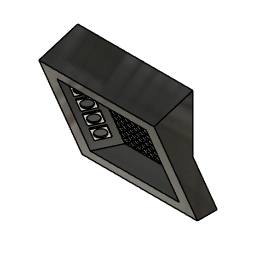
Face (Autodesk Fusion 360 design; units mm, degrees)
Autodesk Fusion 360 part; units mm, degrees
(part 1 of 2)
sketch "Sketch1" plane through (0, 0, 0) normal (0, 1, 0) x (1, 0, 0)
  line L0 (44, 44) -> (-44, 44)
  line L1 (-44, 44) -> (-44, -44)
  line L2 (-44, -44) -> (44, -44)
  line L3 (44, -44) -> (44, 44)
  line L4 (44, 44) -> (-44, -44) construction
  line L5 (-44, 44) -> (44, -44) construction
  dimension "d1" = 88
  dimension "d2" = 88
  constraint horizontal L0
  constraint perpendicular L0 L1
  constraint parallel L0 L2
  constraint parallel L1 L3
  constraint coincident L4 origin
  constraint coincident L5 origin
  measures "d1" distance of L1.end L2.end
  measures "d2" distance of L0.end L1.end
extrude "Extrude1" add sketch "Sketch1" along normal blind 31
sketch "Sketch2" plane through (44, 0, 0) normal (1, 0, 0) x (0, 1, 0)
  line L0 (0, 44) -> (0, -44)
  line L1 (0, -44) -> (31, -44)
  line L2 (31, -44) -> (31, 44)
  line L3 (31, 44) -> (0, 44)
  line L4 (31, 44) -> (31, 0)
  line L5 (31, 0) -> (49.4592, -44)
  line L6 (49.4592, -44) -> (34.4592, -44)
  line L7 (31, 44) -> (1.3859, 34.8347)
  line L8 (1.3859, 34.8347) -> (34.4592, -44)
  dimension "d5" = 15
  dimension "d6" = 31
  constraint coincident L2.end L3.start
  constraint midpoint L2 L4.end
  constraint perpendicular L2 L6
  constraint parallel L5 L8
  constraint collinear L1 L6
  measures "d5" distance of L5.end L6.end
  measures "d6" distance of L2.end L7.end
extrude "Extrude2" cut sketch "Sketch2" against normal blind 88 contours L0 L1 L2 L3 L7 L8
extrude "Extrude3" add sketch "Sketch2" against normal blind 88 contours L2 L5 L6 L8
sketch "Sketch3" plane through (0, 13.6054, 5.7078) normal (0, -0.922137, -0.386863) x (1, 0, 0)
  line L0 (44, -53.905) -> (44, 31.5863)
  line L1 (44, 31.5863) -> (-44, 31.5863)
  line L2 (-44, 31.5863) -> (-44, -53.905)
  line L3 (-44, -53.905) -> (44, -53.905)
  line L4 (34, -43.905) -> (34, 21.5863)
  line L5 (34, 21.5863) -> (-34, 21.5863)
  line L6 (-34, 21.5863) -> (-34, -43.905)
  line L7 (-34, -43.905) -> (34, -43.905)
  dimension "d11" = -10
extrude "Extrude4" cut sketch "Sketch3" against normal blind 80 contours L4 L5 L6 L7
sketch "Sketch4" plane through (0, 16.9852, -40.4865) normal (0, -0.386863, 0.922137) x (1, 0, 0)
  line L0 (34, 28.5863) -> (-34, 28.5863)
  line L1 (-34, 28.5863) -> (-34, 14.7542)
  line L2 (-34, 14.7542) -> (34, 14.7542)
  line L3 (34, 14.7542) -> (34, 28.5863)
  line L4 (-34, 14.7542) -> (-20.1679, 28.5863)
  line L5 (-34, 14.7542) -> (-19.9723, 14.7542) construction
  line L6 (-20.1679, 28.5863) -> (-34, 28.5863)
  line L7 (34, 14.7542) -> (20.1679, 28.5863)
  line L8 (34, 14.7542) -> (60.9464, 14.7542) construction
  line L9 (20.1679, 28.5863) -> (34, 28.5863)
  dimension "d14" = 45
  dimension "d15" = 135
  constraint horizontal L5
  constraint coincident L1.end L2.start
  constraint coincident L0 L4.end
  constraint coincident L0.end L1.start
  constraint horizontal L8
  constraint coincident L2.end L3.start
  constraint coincident L0.start L3.end
  constraint collinear L0 L9
  measures "d14" angle of L4 L5
  measures "d15" angle of L7 L8
extrude "Extrude5" add sketch "Sketch4" along normal up to surface (65.4913 mm away) contours L0 L3 L7 L9 | L0 L1 L4 L6
sketch "Sketch5" plane through (-24.3771, 22.479, 9.4306) normal (0.707107, -0.65205, -0.273553) x (0.677907, 0.735148, 0)
  line L0 (-0.4323, 22.3878) -> (-19.186, 16.8245)
  line L1 (-19.186, 16.8245) -> (-0.5602, -45.9624)
  line L2 (-0.5602, -45.9624) -> (18.1935, -40.3991)
  line L3 (18.1935, -40.3991) -> (-0.4323, 22.3878)
  line L4 (-9.8092, 19.6062) -> (8.8166, -43.1807) construction
  circle A0 centre (4.835, -29.7588) radius 4
  line L5 (-1.3805, -26.3873) -> (8.2065, -23.5433)
  line L6 (8.2065, -23.5433) -> (11.0505, -33.1304)
  line L7 (11.0505, -33.1304) -> (1.4635, -35.9744)
  line L8 (1.4635, -35.9744) -> (-1.3805, -26.3873)
  circle A1 centre (1.043, -16.9761) radius 4
  line L9 (-5.1725, -13.6046) -> (4.4145, -10.7606)
  line L10 (4.4145, -10.7606) -> (7.2585, -20.3476)
  line L11 (7.2585, -20.3476) -> (-2.3285, -23.1916)
  line L12 (-2.3285, -23.1916) -> (-5.1725, -13.6046)
  circle A2 centre (-2.749, -4.1934) radius 4
  line L13 (-8.9646, -0.8218) -> (0.6225, 2.0222)
  line L14 (0.6225, 2.0222) -> (3.4665, -7.5649)
  line L15 (3.4665, -7.5649) -> (-6.1205, -10.4089)
  line L16 (-6.1205, -10.4089) -> (-8.9646, -0.8218)
  circle A3 centre (-6.541, 8.5894) radius 4
  line L17 (-12.7566, 11.9609) -> (-3.1695, 14.8049)
  line L18 (-3.1695, 14.8049) -> (-0.3255, 5.2179)
  line L19 (-0.3255, 5.2179) -> (-9.9126, 2.3739)
  line L20 (-9.9126, 2.3739) -> (-12.7566, 11.9609)
  dimension "d18" = 8
  dimension "d19" = 10
  dimension "d20" = 10
  dimension "d21" = 5
  dimension "d22" = 5
  dimension "d23" = 14
  dimension "d26" = -40
  dimension "d27" = 0
  constraint midpoint L0 L4.start
  constraint midpoint L2 L4.end
  constraint coincident L4 A0.centre
  constraint perpendicular L5 L6
  constraint parallel L5 L7
  constraint parallel L6 L8
  constraint parallel L2 L7
  measures "d18" diameter of A0
  measures "d19" distance of L5.end L6.end
  measures "d20" distance of L6.end L7.end
  measures "d21" distance of A0.centre L6
  measures "d22" distance of A0.centre L7
  measures "d23" distance of L4.end A0.centre
extrude "Extrude6" add sketch "Sketch5" along normal blind 1 contours L5 L6 L7 L8 | L9 L10 L11 L12 | L13 L14 L15 L16 | L17 L18 L19 L20
mirror "Mirror1" about plane through (0, 0, 0) normal (1, 0, 0) of "Extrude6"
sketch "Sketch6" plane through (0, 26.3605, 11.059) normal (0, 0.922137, 0.386863) x (-1, 0, 0)
  line L0 (-34, -11.9927) -> (-44, -11.9927)
  line L1 (-44, -11.9927) -> (-44, -59.708)
  line L2 (-44, -59.708) -> (44, -59.708)
  line L3 (44, -59.708) -> (44, -11.9927)
  line L4 (44, -11.9927) -> (34, -11.9927)
  line L5 (34, -11.9927) -> (34, 21.5863)
  line L6 (34, 21.5863) -> (20.1679, 21.5863)
  line L7 (20.1679, 21.5863) -> (20.1679, -43.905)
  line L8 (20.1679, -43.905) -> (-20.1679, -43.905)
  line L9 (-20.1679, -43.905) -> (-20.1679, 21.5863)
  line L10 (-20.1679, 21.5863) -> (-34, 21.5863)
  line L11 (-34, 21.5863) -> (-34, -11.9927)
  line L12 (-27.084, 21.5863) -> (32.8322, 21.5863)
  line L13 (32.8322, 21.5863) -> (32.8322, -55.186)
  line L14 (32.8322, -55.186) -> (-27.084, -55.186)
  line L15 (-27.084, -55.186) -> (-27.084, 21.5863)
  line L16 (-27, -51.1716) -> (-28.1716, -50)
  line L17 (-28.1716, -50) -> (-29.8284, -50)
  line L18 (-29.8284, -50) -> (-31, -51.1716)
  line L19 (-31, -51.1716) -> (-31, -52.8284)
  line L20 (-31, -52.8284) -> (-29.8284, -54)
  line L21 (-29.8284, -54) -> (-28.1716, -54)
  line L22 (-28.1716, -54) -> (-27, -52.8284)
  line L23 (-27, -52.8284) -> (-27, -51.1716)
  line L24 (-29.8284, -49) -> (-28.1716, -49)
  line L25 (-28.1716, -45) -> (-29.8284, -45)
  line L26 (-28.1716, -49) -> (-27, -47.8284)
  line L27 (-31, -47.8284) -> (-29.8284, -49)
  line L28 (-31, -46.1716) -> (-31, -47.8284)
  line L29 (-27, -47.8284) -> (-27, -46.1716)
  line L30 (-29.8284, -45) -> (-31, -46.1716)
  line L31 (-27, -46.1716) -> (-28.1716, -45)
  line L32 (-29.8284, -44) -> (-28.1716, -44)
  line L33 (-28.1716, -40) -> (-29.8284, -40)
  line L34 (-28.1716, -44) -> (-27, -42.8284)
  line L35 (-31, -42.8284) -> (-29.8284, -44)
  line L36 (-31, -41.1716) -> (-31, -42.8284)
  line L37 (-27, -42.8284) -> (-27, -41.1716)
  line L38 (-29.8284, -40) -> (-31, -41.1716)
  line L39 (-27, -41.1716) -> (-28.1716, -40)
  line L40 (-29.8284, -39) -> (-28.1716, -39)
  line L41 (-28.1716, -35) -> (-29.8284, -35)
  line L42 (-28.1716, -39) -> (-27, -37.8284)
  line L43 (-31, -37.8284) -> (-29.8284, -39)
  line L44 (-31, -36.1716) -> (-31, -37.8284)
  line L45 (-27, -37.8284) -> (-27, -36.1716)
  line L46 (-29.8284, -35) -> (-31, -36.1716)
  line L47 (-27, -36.1716) -> (-28.1716, -35)
  line L48 (-29.8284, -34) -> (-28.1716, -34)
  line L49 (-28.1716, -30) -> (-29.8284, -30)
  line L50 (-28.1716, -34) -> (-27, -32.8284)
  line L51 (-31, -32.8284) -> (-29.8284, -34)
  line L52 (-31, -31.1716) -> (-31, -32.8284)
  line L53 (-27, -32.8284) -> (-27, -31.1716)
  line L54 (-29.8284, -30) -> (-31, -31.1716)
  line L55 (-27, -31.1716) -> (-28.1716, -30)
  line L56 (-29.8284, -29) -> (-28.1716, -29)
  line L57 (-28.1716, -25) -> (-29.8284, -25)
  line L58 (-28.1716, -29) -> (-27, -27.8284)
  line L59 (-31, -27.8284) -> (-29.8284, -29)
  line L60 (-31, -26.1716) -> (-31, -27.8284)
  line L61 (-27, -27.8284) -> (-27, -26.1716)
  line L62 (-29.8284, -25) -> (-31, -26.1716)
  line L63 (-27, -26.1716) -> (-28.1716, -25)
  line L64 (-29.8284, -24) -> (-28.1716, -24)
  line L65 (-28.1716, -20) -> (-29.8284, -20)
  line L66 (-28.1716, -24) -> (-27, -22.8284)
  line L67 (-31, -22.8284) -> (-29.8284, -24)
  line L68 (-31, -21.1716) -> (-31, -22.8284)
  line L69 (-27, -22.8284) -> (-27, -21.1716)
  line L70 (-29.8284, -20) -> (-31, -21.1716)
  line L71 (-27, -21.1716) -> (-28.1716, -20)
  line L72 (-29.8284, -19) -> (-28.1716, -19)
  line L73 (-28.1716, -15) -> (-29.8284, -15)
  line L74 (-28.1716, -19) -> (-27, -17.8284)
  line L75 (-31, -17.8284) -> (-29.8284, -19)
  line L76 (-31, -16.1716) -> (-31, -17.8284)
  line L77 (-27, -17.8284) -> (-27, -16.1716)
  line L78 (-29.8284, -15) -> (-31, -16.1716)
  line L79 (-27, -16.1716) -> (-28.1716, -15)
  line L80 (-29.8284, -14) -> (-28.1716, -14)
  line L81 (-28.1716, -10) -> (-29.8284, -10)
  line L82 (-28.1716, -14) -> (-27, -12.8284)
  line L83 (-31, -12.8284) -> (-29.8284, -14)
  line L84 (-31, -11.1716) -> (-31, -12.8284)
  line L85 (-27, -12.8284) -> (-27, -11.1716)
  line L86 (-29.8284, -10) -> (-31, -11.1716)
  line L87 (-27, -11.1716) -> (-28.1716, -10)
  line L88 (-29.8284, -9) -> (-28.1716, -9)
  line L89 (-28.1716, -5) -> (-29.8284, -5)
  line L90 (-28.1716, -9) -> (-27, -7.8284)
  line L91 (-31, -7.8284) -> (-29.8284, -9)
  line L92 (-31, -6.1716) -> (-31, -7.8284)
  line L93 (-27, -7.8284) -> (-27, -6.1716)
  line L94 (-29.8284, -5) -> (-31, -6.1716)
  line L95 (-27, -6.1716) -> (-28.1716, -5)
  line L96 (-29.8284, -4) -> (-28.1716, -4)
  line L97 (-28.1716, 0) -> (-29.8284, 0)
  line L98 (-28.1716, -4) -> (-27, -2.8284)
  line L99 (-31, -2.8284) -> (-29.8284, -4)
  line L100 (-31, -1.1716) -> (-31, -2.8284)
  line L101 (-27, -2.8284) -> (-27, -1.1716)
  line L102 (-29.8284, 0) -> (-31, -1.1716)
  line L103 (-27, -1.1716) -> (-28.1716, 0)
  line L104 (-29.8284, 1) -> (-28.1716, 1)
  line L105 (-28.1716, 5) -> (-29.8284, 5)
  line L106 (-28.1716, 1) -> (-27, 2.1716)
  line L107 (-31, 2.1716) -> (-29.8284, 1)
  line L108 (-31, 3.8284) -> (-31, 2.1716)
  line L109 (-27, 2.1716) -> (-27, 3.8284)
  line L110 (-29.8284, 5) -> (-31, 3.8284)
  line L111 (-27, 3.8284) -> (-28.1716, 5)
  line L112 (-29.8284, 6) -> (-28.1716, 6)
  line L113 (-28.1716, 10) -> (-29.8284, 10)
  line L114 (-28.1716, 6) -> (-27, 7.1716)
  line L115 (-31, 7.1716) -> (-29.8284, 6)
  line L116 (-31, 8.8284) -> (-31, 7.1716)
  line L117 (-27, 7.1716) -> (-27, 8.8284)
  line L118 (-29.8284, 10) -> (-31, 8.8284)
  line L119 (-27, 8.8284) -> (-28.1716, 10)
  line L120 (-29.8284, 11) -> (-28.1716, 11)
  line L121 (-28.1716, 15) -> (-29.8284, 15)
  line L122 (-28.1716, 11) -> (-27, 12.1716)
  line L123 (-31, 12.1716) -> (-29.8284, 11)
  line L124 (-31, 13.8284) -> (-31, 12.1716)
  line L125 (-27, 12.1716) -> (-27, 13.8284)
  line L126 (-29.8284, 15) -> (-31, 13.8284)
  line L127 (-27, 13.8284) -> (-28.1716, 15)
  line L128 (-29.8284, 16) -> (-28.1716, 16)
  line L129 (-28.1716, 20) -> (-29.8284, 20)
  line L130 (-28.1716, 16) -> (-27, 17.1716)
  line L131 (-31, 17.1716) -> (-29.8284, 16)
  line L132 (-31, 18.8284) -> (-31, 17.1716)
  line L133 (-27, 17.1716) -> (-27, 18.8284)
  line L134 (-29.8284, 20) -> (-31, 18.8284)
  line L135 (-27, 18.8284) -> (-28.1716, 20)
  line L136 (-26.0833, -6.1716) -> (-26.0833, -7.8284)
  line L137 (-23.2549, -40) -> (-24.9118, -40)
  line L138 (-22.0833, -27.8284) -> (-22.0833, -26.1716)
  line L139 (-24.9118, 5) -> (-26.0833, 3.8284)
  line L140 (-26.0833, -31.1716) -> (-26.0833, -32.8284)
  line L141 (-22.0833, -2.8284) -> (-22.0833, -1.1716)
  line L142 (-24.9118, 20) -> (-26.0833, 18.8284)
  line L143 (-26.0833, 2.1716) -> (-24.9118, 1)
  line L144 (-26.0833, -1.1716) -> (-26.0833, -2.8284)
  line L145 (-26.0833, 18.8284) -> (-26.0833, 17.1716)
  line L146 (-24.9118, -29) -> (-23.2549, -29)
  line L147 (-23.2549, -49) -> (-22.0833, -47.8284)
  line L148 (-23.2549, 5) -> (-24.9118, 5)
  line L149 (-23.2549, -24) -> (-22.0833, -22.8284)
  line L150 (-26.0833, -51.1716) -> (-26.0833, -52.8284)
  line L151 (-22.0833, -6.1716) -> (-23.2549, -5)
  line L152 (-22.0833, -47.8284) -> (-22.0833, -46.1716)
  line L153 (-22.0833, -32.8284) -> (-22.0833, -31.1716)
  line L154 (-22.0833, 8.8284) -> (-23.2549, 10)
  line L155 (-26.0833, 17.1716) -> (-24.9118, 16)
  line L156 (-24.9118, -9) -> (-23.2549, -9)
  line L157 (-22.0833, -46.1716) -> (-23.2549, -45)
  line L158 (-23.2549, 16) -> (-22.0833, 17.1716)
  line L159 (-23.2549, -44) -> (-22.0833, -42.8284)
  line L160 (-24.9118, -14) -> (-23.2549, -14)
  line L161 (-23.2549, 6) -> (-22.0833, 7.1716)
  line L162 (-24.9118, -49) -> (-23.2549, -49)
  line L163 (-24.9118, -44) -> (-23.2549, -44)
  line L164 (-22.0833, -21.1716) -> (-23.2549, -20)
  line L165 (-24.9118, 1) -> (-23.2549, 1)
  line L166 (-23.2549, -4) -> (-22.0833, -2.8284)
  line L167 (-22.0833, -17.8284) -> (-22.0833, -16.1716)
  line L168 (-23.2549, -30) -> (-24.9118, -30)
  line L169 (-24.9118, -5) -> (-26.0833, -6.1716)
  line L170 (-23.2549, -19) -> (-22.0833, -17.8284)
  line L171 (-23.2549, -14) -> (-22.0833, -12.8284)
  line L172 (-26.0833, -22.8284) -> (-24.9118, -24)
  line L173 (-23.2549, -34) -> (-22.0833, -32.8284)
  line L174 (-22.0833, -31.1716) -> (-23.2549, -30)
  line L175 (-22.0833, -12.8284) -> (-22.0833, -11.1716)
  line L176 (-26.0833, -21.1716) -> (-26.0833, -22.8284)
  line L177 (-24.9118, -35) -> (-26.0833, -36.1716)
  line L178 (-24.9118, 0) -> (-26.0833, -1.1716)
  line L179 (-26.0833, -52.8284) -> (-24.9118, -54)
  line L180 (-23.2549, -10) -> (-24.9118, -10)
  line L181 (-23.2549, 1) -> (-22.0833, 2.1716)
  line L182 (-26.0833, -17.8284) -> (-24.9118, -19)
  line L183 (-26.0833, -46.1716) -> (-26.0833, -47.8284)
  line L184 (-22.0833, 17.1716) -> (-22.0833, 18.8284)
  line L185 (-24.9118, -19) -> (-23.2549, -19)
  line L186 (-24.9118, 16) -> (-23.2549, 16)
  line L187 (-24.9118, 6) -> (-23.2549, 6)
  line L188 (-24.9118, -24) -> (-23.2549, -24)
  line L189 (-24.9118, -25) -> (-26.0833, -26.1716)
  line L190 (-23.2549, -35) -> (-24.9118, -35)
  line L191 (-22.0833, 12.1716) -> (-22.0833, 13.8284)
  line L192 (-23.2549, -50) -> (-24.9118, -50)
  line L193 (-26.0833, 8.8284) -> (-26.0833, 7.1716)
  line L194 (-23.2549, 15) -> (-24.9118, 15)
  line L195 (-23.2549, -45) -> (-24.9118, -45)
  line L196 (-23.2549, 10) -> (-24.9118, 10)
  line L197 (-26.0833, -7.8284) -> (-24.9118, -9)
  line L198 (-24.9118, -50) -> (-26.0833, -51.1716)
  line L199 (-22.0833, -36.1716) -> (-23.2549, -35)
  line L200 (-26.0833, 13.8284) -> (-26.0833, 12.1716)
  line L201 (-23.2549, -9) -> (-22.0833, -7.8284)
  line L202 (-24.9118, -20) -> (-26.0833, -21.1716)
  line L203 (-24.9118, -10) -> (-26.0833, -11.1716)
  line L204 (-26.0833, -41.1716) -> (-26.0833, -42.8284)
  line L205 (-26.0833, 7.1716) -> (-24.9118, 6)
  line L206 (-24.9118, -15) -> (-26.0833, -16.1716)
  line L207 (-26.0833, -32.8284) -> (-24.9118, -34)
  line L208 (-26.0833, -42.8284) -> (-24.9118, -44)
  line L209 (-23.2549, -25) -> (-24.9118, -25)
  line L210 (-26.0833, -47.8284) -> (-24.9118, -49)
  line L211 (-22.0833, -26.1716) -> (-23.2549, -25)
  line L212 (-24.9118, -39) -> (-23.2549, -39)
  line L213 (-23.2549, 0) -> (-24.9118, 0)
  line L214 (-24.9118, 15) -> (-26.0833, 13.8284)
  line L215 (-26.0833, -37.8284) -> (-24.9118, -39)
  line L216 (-23.2549, -20) -> (-24.9118, -20)
  line L217 (-24.9118, 11) -> (-23.2549, 11)
  line L218 (-22.0833, -11.1716) -> (-23.2549, -10)
  line L219 (-26.0833, -27.8284) -> (-24.9118, -29)
  line L220 (-24.9118, 10) -> (-26.0833, 8.8284)
  line L221 (-23.2549, 11) -> (-22.0833, 12.1716)
  line L222 (-22.0833, -1.1716) -> (-23.2549, 0)
  line L223 (-23.2549, -39) -> (-22.0833, -37.8284)
  line L224 (-24.9118, -45) -> (-26.0833, -46.1716)
  line L225 (-22.0833, -22.8284) -> (-22.0833, -21.1716)
  line L226 (-26.0833, -26.1716) -> (-26.0833, -27.8284)
  line L227 (-26.0833, -16.1716) -> (-26.0833, -17.8284)
  line L228 (-23.2549, -54) -> (-22.0833, -52.8284)
  line L229 (-22.0833, -16.1716) -> (-23.2549, -15)
  line L230 (-26.0833, -11.1716) -> (-26.0833, -12.8284)
  line L231 (-24.9118, -40) -> (-26.0833, -41.1716)
  line L232 (-26.0833, -2.8284) -> (-24.9118, -4)
  line L233 (-26.0833, -12.8284) -> (-24.9118, -14)
  line L234 (-26.0833, 3.8284) -> (-26.0833, 2.1716)
  line L235 (-22.0833, -37.8284) -> (-22.0833, -36.1716)
  line L236 (-22.0833, -52.8284) -> (-22.0833, -51.1716)
  line L237 (-22.0833, -42.8284) -> (-22.0833, -41.1716)
  line L238 (-22.0833, 3.8284) -> (-23.2549, 5)
  line L239 (-23.2549, -5) -> (-24.9118, -5)
  line L240 (-22.0833, -51.1716) -> (-23.2549, -50)
  line L241 (-24.9118, -30) -> (-26.0833, -31.1716)
  line L242 (-24.9118, -4) -> (-23.2549, -4)
  line L243 (-22.0833, 7.1716) -> (-22.0833, 8.8284)
  line L244 (-24.9118, -34) -> (-23.2549, -34)
  line L245 (-23.2549, -15) -> (-24.9118, -15)
  line L246 (-22.0833, 2.1716) -> (-22.0833, 3.8284)
  line L247 (-23.2549, 20) -> (-24.9118, 20)
  line L248 (-24.9118, -54) -> (-23.2549, -54)
  line L249 (-26.0833, 12.1716) -> (-24.9118, 11)
  line L250 (-26.0833, -36.1716) -> (-26.0833, -37.8284)
  line L251 (-22.0833, -41.1716) -> (-23.2549, -40)
  line L252 (-22.0833, 13.8284) -> (-23.2549, 15)
  line L253 (-22.0833, 18.8284) -> (-23.2549, 20)
  line L254 (-22.0833, -7.8284) -> (-22.0833, -6.1716)
  line L255 (-23.2549, -29) -> (-22.0833, -27.8284)
  line L256 (-21.1667, -6.1716) -> (-21.1667, -7.8284)
  line L257 (-18.3382, -40) -> (-19.9951, -40)
  line L258 (-17.1667, -27.8284) -> (-17.1667, -26.1716)
  line L259 (-19.9951, 5) -> (-21.1667, 3.8284)
  line L260 (-21.1667, -31.1716) -> (-21.1667, -32.8284)
  line L261 (-17.1667, -2.8284) -> (-17.1667, -1.1716)
  line L262 (-19.9951, 20) -> (-21.1667, 18.8284)
  line L263 (-21.1667, 2.1716) -> (-19.9951, 1)
  line L264 (-21.1667, -1.1716) -> (-21.1667, -2.8284)
  line L265 (-21.1667, 18.8284) -> (-21.1667, 17.1716)
  line L266 (-19.9951, -29) -> (-18.3382, -29)
  line L267 (-18.3382, -49) -> (-17.1667, -47.8284)
  line L268 (-18.3382, 5) -> (-19.9951, 5)
  line L269 (-18.3382, -24) -> (-17.1667, -22.8284)
  line L270 (-21.1667, -51.1716) -> (-21.1667, -52.8284)
  line L271 (-17.1667, -6.1716) -> (-18.3382, -5)
  line L272 (-17.1667, -47.8284) -> (-17.1667, -46.1716)
  line L273 (-17.1667, -32.8284) -> (-17.1667, -31.1716)
  line L274 (-17.1667, 8.8284) -> (-18.3382, 10)
  line L275 (-21.1667, 17.1716) -> (-19.9951, 16)
  line L276 (-19.9951, -9) -> (-18.3382, -9)
  line L277 (-17.1667, -46.1716) -> (-18.3382, -45)
  line L278 (-18.3382, 16) -> (-17.1667, 17.1716)
  line L279 (-18.3382, -44) -> (-17.1667, -42.8284)
  line L280 (-19.9951, -14) -> (-18.3382, -14)
  line L281 (-18.3382, 6) -> (-17.1667, 7.1716)
  line L282 (-19.9951, -49) -> (-18.3382, -49)
  line L283 (-19.9951, -44) -> (-18.3382, -44)
  line L284 (-17.1667, -21.1716) -> (-18.3382, -20)
  line L285 (-19.9951, 1) -> (-18.3382, 1)
  line L286 (-18.3382, -4) -> (-17.1667, -2.8284)
  line L287 (-17.1667, -17.8284) -> (-17.1667, -16.1716)
  line L288 (-18.3382, -30) -> (-19.9951, -30)
  line L289 (-19.9951, -5) -> (-21.1667, -6.1716)
  line L290 (-18.3382, -19) -> (-17.1667, -17.8284)
  line L291 (-18.3382, -14) -> (-17.1667, -12.8284)
  line L292 (-21.1667, -22.8284) -> (-19.9951, -24)
  line L293 (-18.3382, -34) -> (-17.1667, -32.8284)
  line L294 (-17.1667, -31.1716) -> (-18.3382, -30)
  line L295 (-17.1667, -12.8284) -> (-17.1667, -11.1716)
  line L296 (-21.1667, -21.1716) -> (-21.1667, -22.8284)
  line L297 (-19.9951, -35) -> (-21.1667, -36.1716)
  line L298 (-19.9951, 0) -> (-21.1667, -1.1716)
  line L299 (-21.1667, -52.8284) -> (-19.9951, -54)
  line L300 (-18.3382, -10) -> (-19.9951, -10)
  line L301 (-18.3382, 1) -> (-17.1667, 2.1716)
  line L302 (-21.1667, -17.8284) -> (-19.9951, -19)
  line L303 (-21.1667, -46.1716) -> (-21.1667, -47.8284)
  line L304 (-17.1667, 17.1716) -> (-17.1667, 18.8284)
  line L305 (-19.9951, -19) -> (-18.3382, -19)
  line L306 (-19.9951, 16) -> (-18.3382, 16)
  line L307 (-19.9951, 6) -> (-18.3382, 6)
  line L308 (-19.9951, -24) -> (-18.3382, -24)
  line L309 (-19.9951, -25) -> (-21.1667, -26.1716)
  line L310 (-18.3382, -35) -> (-19.9951, -35)
  line L311 (-17.1667, 12.1716) -> (-17.1667, 13.8284)
  line L312 (-18.3382, -50) -> (-19.9951, -50)
  line L313 (-21.1667, 8.8284) -> (-21.1667, 7.1716)
  line L314 (-18.3382, 15) -> (-19.9951, 15)
  line L315 (-18.3382, -45) -> (-19.9951, -45)
  line L316 (-18.3382, 10) -> (-19.9951, 10)
  line L317 (-21.1667, -7.8284) -> (-19.9951, -9)
  line L318 (-19.9951, -50) -> (-21.1667, -51.1716)
  line L319 (-17.1667, -36.1716) -> (-18.3382, -35)
  line L320 (-21.1667, 13.8284) -> (-21.1667, 12.1716)
  line L321 (-18.3382, -9) -> (-17.1667, -7.8284)
  line L322 (-19.9951, -20) -> (-21.1667, -21.1716)
  line L323 (-19.9951, -10) -> (-21.1667, -11.1716)
  line L324 (-21.1667, -41.1716) -> (-21.1667, -42.8284)
  line L325 (-21.1667, 7.1716) -> (-19.9951, 6)
  line L326 (-19.9951, -15) -> (-21.1667, -16.1716)
  line L327 (-21.1667, -32.8284) -> (-19.9951, -34)
  line L328 (-21.1667, -42.8284) -> (-19.9951, -44)
  line L329 (-18.3382, -25) -> (-19.9951, -25)
  line L330 (-21.1667, -47.8284) -> (-19.9951, -49)
  line L331 (-17.1667, -26.1716) -> (-18.3382, -25)
  line L332 (-19.9951, -39) -> (-18.3382, -39)
  line L333 (-18.3382, 0) -> (-19.9951, 0)
  line L334 (-19.9951, 15) -> (-21.1667, 13.8284)
  line L335 (-21.1667, -37.8284) -> (-19.9951, -39)
  line L336 (-18.3382, -20) -> (-19.9951, -20)
  line L337 (-19.9951, 11) -> (-18.3382, 11)
  line L338 (-17.1667, -11.1716) -> (-18.3382, -10)
  line L339 (-21.1667, -27.8284) -> (-19.9951, -29)
  line L340 (-19.9951, 10) -> (-21.1667, 8.8284)
  line L341 (-18.3382, 11) -> (-17.1667, 12.1716)
  line L342 (-17.1667, -1.1716) -> (-18.3382, 0)
  line L343 (-18.3382, -39) -> (-17.1667, -37.8284)
  line L344 (-19.9951, -45) -> (-21.1667, -46.1716)
  line L345 (-17.1667, -22.8284) -> (-17.1667, -21.1716)
  line L346 (-21.1667, -26.1716) -> (-21.1667, -27.8284)
  line L347 (-21.1667, -16.1716) -> (-21.1667, -17.8284)
  line L348 (-18.3382, -54) -> (-17.1667, -52.8284)
  line L349 (-17.1667, -16.1716) -> (-18.3382, -15)
  line L350 (-21.1667, -11.1716) -> (-21.1667, -12.8284)
  line L351 (-19.9951, -40) -> (-21.1667, -41.1716)
  line L352 (-21.1667, -2.8284) -> (-19.9951, -4)
  line L353 (-21.1667, -12.8284) -> (-19.9951, -14)
  line L354 (-21.1667, 3.8284) -> (-21.1667, 2.1716)
  line L355 (-17.1667, -37.8284) -> (-17.1667, -36.1716)
  line L356 (-17.1667, -52.8284) -> (-17.1667, -51.1716)
  line L357 (-17.1667, -42.8284) -> (-17.1667, -41.1716)
  line L358 (-17.1667, 3.8284) -> (-18.3382, 5)
  line L359 (-18.3382, -5) -> (-19.9951, -5)
  line L360 (-17.1667, -51.1716) -> (-18.3382, -50)
  line L361 (-19.9951, -30) -> (-21.1667, -31.1716)
  line L362 (-19.9951, -4) -> (-18.3382, -4)
  line L363 (-17.1667, 7.1716) -> (-17.1667, 8.8284)
  line L364 (-19.9951, -34) -> (-18.3382, -34)
  line L365 (-18.3382, -15) -> (-19.9951, -15)
  line L366 (-17.1667, 2.1716) -> (-17.1667, 3.8284)
  line L367 (-18.3382, 20) -> (-19.9951, 20)
  line L368 (-19.9951, -54) -> (-18.3382, -54)
  line L369 (-21.1667, 12.1716) -> (-19.9951, 11)
  line L370 (-21.1667, -36.1716) -> (-21.1667, -37.8284)
  line L371 (-17.1667, -41.1716) -> (-18.3382, -40)
  line L372 (-17.1667, 13.8284) -> (-18.3382, 15)
  line L373 (-17.1667, 18.8284) -> (-18.3382, 20)
  line L374 (-17.1667, -7.8284) -> (-17.1667, -6.1716)
  line L375 (-18.3382, -29) -> (-17.1667, -27.8284)
  line L376 (-16.25, -6.1716) -> (-16.25, -7.8284)
  line L377 (-13.4216, -40) -> (-15.0784, -40)
  line L378 (-12.25, -27.8284) -> (-12.25, -26.1716)
  line L379 (-15.0784, 5) -> (-16.25, 3.8284)
  line L380 (-16.25, -31.1716) -> (-16.25, -32.8284)
  line L381 (-12.25, -2.8284) -> (-12.25, -1.1716)
  line L382 (-15.0784, 20) -> (-16.25, 18.8284)
  line L383 (-16.25, 2.1716) -> (-15.0784, 1)
  line L384 (-16.25, -1.1716) -> (-16.25, -2.8284)
  line L385 (-16.25, 18.8284) -> (-16.25, 17.1716)
  line L386 (-15.0784, -29) -> (-13.4216, -29)
  line L387 (-13.4216, -49) -> (-12.25, -47.8284)
  line L388 (-13.4216, 5) -> (-15.0784, 5)
  line L389 (-13.4216, -24) -> (-12.25, -22.8284)
  line L390 (-16.25, -51.1716) -> (-16.25, -52.8284)
  line L391 (-12.25, -6.1716) -> (-13.4216, -5)
  line L392 (-12.25, -47.8284) -> (-12.25, -46.1716)
  line L393 (-12.25, -32.8284) -> (-12.25, -31.1716)
  line L394 (-12.25, 8.8284) -> (-13.4216, 10)
  line L395 (-16.25, 17.1716) -> (-15.0784, 16)
  line L396 (-15.0784, -9) -> (-13.4216, -9)
  line L397 (-12.25, -46.1716) -> (-13.4216, -45)
  line L398 (-13.4216, 16) -> (-12.25, 17.1716)
  line L399 (-13.4216, -44) -> (-12.25, -42.8284)
  line L400 (-15.0784, -14) -> (-13.4216, -14)
  line L401 (-13.4216, 6) -> (-12.25, 7.1716)
  line L402 (-15.0784, -49) -> (-13.4216, -49)
  line L403 (-15.0784, -44) -> (-13.4216, -44)
  line L404 (-12.25, -21.1716) -> (-13.4216, -20)
  line L405 (-15.0784, 1) -> (-13.4216, 1)
  line L406 (-13.4216, -4) -> (-12.25, -2.8284)
  line L407 (-12.25, -17.8284) -> (-12.25, -16.1716)
  line L408 (-13.4216, -30) -> (-15.0784, -30)
  line L409 (-15.0784, -5) -> (-16.25, -6.1716)
  line L410 (-13.4216, -19) -> (-12.25, -17.8284)
  line L411 (-13.4216, -14) -> (-12.25, -12.8284)
  line L412 (-16.25, -22.8284) -> (-15.0784, -24)
  line L413 (-13.4216, -34) -> (-12.25, -32.8284)
  line L414 (-12.25, -31.1716) -> (-13.4216, -30)
  line L415 (-12.25, -12.8284) -> (-12.25, -11.1716)
  line L416 (-16.25, -21.1716) -> (-16.25, -22.8284)
  line L417 (-15.0784, -35) -> (-16.25, -36.1716)
  line L418 (-15.0784, 0) -> (-16.25, -1.1716)
  line L419 (-16.25, -52.8284) -> (-15.0784, -54)
  line L420 (-13.4216, -10) -> (-15.0784, -10)
  line L421 (-13.4216, 1) -> (-12.25, 2.1716)
  line L422 (-16.25, -17.8284) -> (-15.0784, -19)
  line L423 (-16.25, -46.1716) -> (-16.25, -47.8284)
  line L424 (-12.25, 17.1716) -> (-12.25, 18.8284)
  line L425 (-15.0784, -19) -> (-13.4216, -19)
  line L426 (-15.0784, 16) -> (-13.4216, 16)
  line L427 (-15.0784, 6) -> (-13.4216, 6)
  line L428 (-15.0784, -24) -> (-13.4216, -24)
  line L429 (-15.0784, -25) -> (-16.25, -26.1716)
  line L430 (-13.4216, -35) -> (-15.0784, -35)
  line L431 (-12.25, 12.1716) -> (-12.25, 13.8284)
  line L432 (-13.4216, -50) -> (-15.0784, -50)
  line L433 (-16.25, 8.8284) -> (-16.25, 7.1716)
  line L434 (-13.4216, 15) -> (-15.0784, 15)
  line L435 (-13.4216, -45) -> (-15.0784, -45)
  line L436 (-13.4216, 10) -> (-15.0784, 10)
  line L437 (-16.25, -7.8284) -> (-15.0784, -9)
  line L438 (-15.0784, -50) -> (-16.25, -51.1716)
  line L439 (-12.25, -36.1716) -> (-13.4216, -35)
  line L440 (-16.25, 13.8284) -> (-16.25, 12.1716)
  line L441 (-13.4216, -9) -> (-12.25, -7.8284)
  line L442 (-15.0784, -20) -> (-16.25, -21.1716)
  line L443 (-15.0784, -10) -> (-16.25, -11.1716)
  line L444 (-16.25, -41.1716) -> (-16.25, -42.8284)
  line L445 (-16.25, 7.1716) -> (-15.0784, 6)
  line L446 (-15.0784, -15) -> (-16.25, -16.1716)
  line L447 (-16.25, -32.8284) -> (-15.0784, -34)
  line L448 (-16.25, -42.8284) -> (-15.0784, -44)
  line L449 (-13.4216, -25) -> (-15.0784, -25)
  line L450 (-16.25, -47.8284) -> (-15.0784, -49)
  line L451 (-12.25, -26.1716) -> (-13.4216, -25)
  line L452 (-15.0784, -39) -> (-13.4216, -39)
  line L453 (-13.4216, 0) -> (-15.0784, 0)
  line L454 (-15.0784, 15) -> (-16.25, 13.8284)
  line L455 (-16.25, -37.8284) -> (-15.0784, -39)
  line L456 (-13.4216, -20) -> (-15.0784, -20)
  line L457 (-15.0784, 11) -> (-13.4216, 11)
  line L458 (-12.25, -11.1716) -> (-13.4216, -10)
  line L459 (-16.25, -27.8284) -> (-15.0784, -29)
  line L460 (-15.0784, 10) -> (-16.25, 8.8284)
  line L461 (-13.4216, 11) -> (-12.25, 12.1716)
  line L462 (-12.25, -1.1716) -> (-13.4216, 0)
  line L463 (-13.4216, -39) -> (-12.25, -37.8284)
  line L464 (-15.0784, -45) -> (-16.25, -46.1716)
  line L465 (-12.25, -22.8284) -> (-12.25, -21.1716)
  line L466 (-16.25, -26.1716) -> (-16.25, -27.8284)
  line L467 (-16.25, -16.1716) -> (-16.25, -17.8284)
  line L468 (-13.4216, -54) -> (-12.25, -52.8284)
  line L469 (-12.25, -16.1716) -> (-13.4216, -15)
  line L470 (-16.25, -11.1716) -> (-16.25, -12.8284)
  line L471 (-15.0784, -40) -> (-16.25, -41.1716)
  line L472 (-16.25, -2.8284) -> (-15.0784, -4)
  line L473 (-16.25, -12.8284) -> (-15.0784, -14)
  line L474 (-16.25, 3.8284) -> (-16.25, 2.1716)
  line L475 (-12.25, -37.8284) -> (-12.25, -36.1716)
  line L476 (-12.25, -52.8284) -> (-12.25, -51.1716)
  line L477 (-12.25, -42.8284) -> (-12.25, -41.1716)
  line L478 (-12.25, 3.8284) -> (-13.4216, 5)
  line L479 (-13.4216, -5) -> (-15.0784, -5)
  line L480 (-12.25, -51.1716) -> (-13.4216, -50)
  line L481 (-15.0784, -30) -> (-16.25, -31.1716)
  line L482 (-15.0784, -4) -> (-13.4216, -4)
  line L483 (-12.25, 7.1716) -> (-12.25, 8.8284)
  line L484 (-15.0784, -34) -> (-13.4216, -34)
  line L485 (-13.4216, -15) -> (-15.0784, -15)
  line L486 (-12.25, 2.1716) -> (-12.25, 3.8284)
  line L487 (-13.4216, 20) -> (-15.0784, 20)
  line L488 (-15.0784, -54) -> (-13.4216, -54)
  line L489 (-16.25, 12.1716) -> (-15.0784, 11)
  line L490 (-16.25, -36.1716) -> (-16.25, -37.8284)
  line L491 (-12.25, -41.1716) -> (-13.4216, -40)
  line L492 (-12.25, 13.8284) -> (-13.4216, 15)
  line L493 (-12.25, 18.8284) -> (-13.4216, 20)
  line L494 (-12.25, -7.8284) -> (-12.25, -6.1716)
  line L495 (-13.4216, -29) -> (-12.25, -27.8284)
  line L496 (-11.3333, -6.1716) -> (-11.3333, -7.8284)
  line L497 (-8.5049, -40) -> (-10.1618, -40)
  line L498 (-7.3333, -27.8284) -> (-7.3333, -26.1716)
  line L499 (-10.1618, 5) -> (-11.3333, 3.8284)
  line L500 (-11.3333, -31.1716) -> (-11.3333, -32.8284)
  line L501 (-7.3333, -2.8284) -> (-7.3333, -1.1716)
  line L502 (-10.1618, 20) -> (-11.3333, 18.8284)
  line L503 (-11.3333, 2.1716) -> (-10.1618, 1)
  line L504 (-11.3333, -1.1716) -> (-11.3333, -2.8284)
  line L505 (-11.3333, 18.8284) -> (-11.3333, 17.1716)
  line L506 (-10.1618, -29) -> (-8.5049, -29)
  line L507 (-8.5049, -49) -> (-7.3333, -47.8284)
  line L508 (-8.5049, 5) -> (-10.1618, 5)
  line L509 (-8.5049, -24) -> (-7.3333, -22.8284)
  line L510 (-11.3333, -51.1716) -> (-11.3333, -52.8284)
  line L511 (-7.3333, -6.1716) -> (-8.5049, -5)
  line L512 (-7.3333, -47.8284) -> (-7.3333, -46.1716)
  line L513 (-7.3333, -32.8284) -> (-7.3333, -31.1716)
  line L514 (-7.3333, 8.8284) -> (-8.5049, 10)
  line L515 (-11.3333, 17.1716) -> (-10.1618, 16)
  line L516 (-10.1618, -9) -> (-8.5049, -9)
  line L517 (-7.3333, -46.1716) -> (-8.5049, -45)
  line L518 (-8.5049, 16) -> (-7.3333, 17.1716)
  line L519 (-8.5049, -44) -> (-7.3333, -42.8284)
  line L520 (-10.1618, -14) -> (-8.5049, -14)
  line L521 (-8.5049, 6) -> (-7.3333, 7.1716)
  line L522 (-10.1618, -49) -> (-8.5049, -49)
  line L523 (-10.1618, -44) -> (-8.5049, -44)
  line L524 (-7.3333, -21.1716) -> (-8.5049, -20)
  line L525 (-10.1618, 1) -> (-8.5049, 1)
  line L526 (-8.5049, -4) -> (-7.3333, -2.8284)
  line L527 (-7.3333, -17.8284) -> (-7.3333, -16.1716)
  line L528 (-8.5049, -30) -> (-10.1618, -30)
  line L529 (-10.1618, -5) -> (-11.3333, -6.1716)
  line L530 (-8.5049, -19) -> (-7.3333, -17.8284)
  line L531 (-8.5049, -14) -> (-7.3333, -12.8284)
  line L532 (-11.3333, -22.8284) -> (-10.1618, -24)
  line L533 (-8.5049, -34) -> (-7.3333, -32.8284)
  line L534 (-7.3333, -31.1716) -> (-8.5049, -30)
  line L535 (-7.3333, -12.8284) -> (-7.3333, -11.1716)
  line L536 (-11.3333, -21.1716) -> (-11.3333, -22.8284)
  line L537 (-10.1618, -35) -> (-11.3333, -36.1716)
  line L538 (-10.1618, 0) -> (-11.3333, -1.1716)
  line L539 (-11.3333, -52.8284) -> (-10.1618, -54)
  line L540 (-8.5049, -10) -> (-10.1618, -10)
  line L541 (-8.5049, 1) -> (-7.3333, 2.1716)
  line L542 (-11.3333, -17.8284) -> (-10.1618, -19)
  line L543 (-11.3333, -46.1716) -> (-11.3333, -47.8284)
  line L544 (-7.3333, 17.1716) -> (-7.3333, 18.8284)
  line L545 (-10.1618, -19) -> (-8.5049, -19)
  line L546 (-10.1618, 16) -> (-8.5049, 16)
  line L547 (-10.1618, 6) -> (-8.5049, 6)
  line L548 (-10.1618, -24) -> (-8.5049, -24)
  line L549 (-10.1618, -25) -> (-11.3333, -26.1716)
  line L550 (-8.5049, -35) -> (-10.1618, -35)
  line L551 (-7.3333, 12.1716) -> (-7.3333, 13.8284)
  line L552 (-8.5049, -50) -> (-10.1618, -50)
  line L553 (-11.3333, 8.8284) -> (-11.3333, 7.1716)
  line L554 (-8.5049, 15) -> (-10.1618, 15)
  line L555 (-8.5049, -45) -> (-10.1618, -45)
  line L556 (-8.5049, 10) -> (-10.1618, 10)
  line L557 (-11.3333, -7.8284) -> (-10.1618, -9)
  line L558 (-10.1618, -50) -> (-11.3333, -51.1716)
  line L559 (-7.3333, -36.1716) -> (-8.5049, -35)
  line L560 (-11.3333, 13.8284) -> (-11.3333, 12.1716)
  line L561 (-8.5049, -9) -> (-7.3333, -7.8284)
  line L562 (-10.1618, -20) -> (-11.3333, -21.1716)
  line L563 (-10.1618, -10) -> (-11.3333, -11.1716)
  line L564 (-11.3333, -41.1716) -> (-11.3333, -42.8284)
  line L565 (-11.3333, 7.1716) -> (-10.1618, 6)
  line L566 (-10.1618, -15) -> (-11.3333, -16.1716)
  line L567 (-11.3333, -32.8284) -> (-10.1618, -34)
  line L568 (-11.3333, -42.8284) -> (-10.1618, -44)
  line L569 (-8.5049, -25) -> (-10.1618, -25)
  line L570 (-11.3333, -47.8284) -> (-10.1618, -49)
  line L571 (-7.3333, -26.1716) -> (-8.5049, -25)
  line L572 (-10.1618, -39) -> (-8.5049, -39)
  line L573 (-8.5049, 0) -> (-10.1618, 0)
  line L574 (-10.1618, 15) -> (-11.3333, 13.8284)
  line L575 (-11.3333, -37.8284) -> (-10.1618, -39)
  line L576 (-8.5049, -20) -> (-10.1618, -20)
  line L577 (-10.1618, 11) -> (-8.5049, 11)
  line L578 (-7.3333, -11.1716) -> (-8.5049, -10)
  line L579 (-11.3333, -27.8284) -> (-10.1618, -29)
  line L580 (-10.1618, 10) -> (-11.3333, 8.8284)
  line L581 (-8.5049, 11) -> (-7.3333, 12.1716)
  line L582 (-7.3333, -1.1716) -> (-8.5049, 0)
  line L583 (-8.5049, -39) -> (-7.3333, -37.8284)
  line L584 (-10.1618, -45) -> (-11.3333, -46.1716)
  line L585 (-7.3333, -22.8284) -> (-7.3333, -21.1716)
  line L586 (-11.3333, -26.1716) -> (-11.3333, -27.8284)
  line L587 (-11.3333, -16.1716) -> (-11.3333, -17.8284)
  line L588 (-8.5049, -54) -> (-7.3333, -52.8284)
  line L589 (-7.3333, -16.1716) -> (-8.5049, -15)
  line L590 (-11.3333, -11.1716) -> (-11.3333, -12.8284)
  line L591 (-10.1618, -40) -> (-11.3333, -41.1716)
  line L592 (-11.3333, -2.8284) -> (-10.1618, -4)
  line L593 (-11.3333, -12.8284) -> (-10.1618, -14)
  line L594 (-11.3333, 3.8284) -> (-11.3333, 2.1716)
  line L595 (-7.3333, -37.8284) -> (-7.3333, -36.1716)
  line L596 (-7.3333, -52.8284) -> (-7.3333, -51.1716)
  line L597 (-7.3333, -42.8284) -> (-7.3333, -41.1716)
  line L598 (-7.3333, 3.8284) -> (-8.5049, 5)
  line L599 (-8.5049, -5) -> (-10.1618, -5)
  line L600 (-7.3333, -51.1716) -> (-8.5049, -50)
  line L601 (-10.1618, -30) -> (-11.3333, -31.1716)
  line L602 (-10.1618, -4) -> (-8.5049, -4)
  line L603 (-7.3333, 7.1716) -> (-7.3333, 8.8284)
  line L604 (-10.1618, -34) -> (-8.5049, -34)
  line L605 (-8.5049, -15) -> (-10.1618, -15)
  line L606 (-7.3333, 2.1716) -> (-7.3333, 3.8284)
  line L607 (-8.5049, 20) -> (-10.1618, 20)
  line L608 (-10.1618, -54) -> (-8.5049, -54)
  line L609 (-11.3333, 12.1716) -> (-10.1618, 11)
  line L610 (-11.3333, -36.1716) -> (-11.3333, -37.8284)
  line L611 (-7.3333, -41.1716) -> (-8.5049, -40)
  line L612 (-7.3333, 13.8284) -> (-8.5049, 15)
  line L613 (-7.3333, 18.8284) -> (-8.5049, 20)
  line L614 (-7.3333, -7.8284) -> (-7.3333, -6.1716)
  line L615 (-8.5049, -29) -> (-7.3333, -27.8284)
  line L616 (-6.4167, -6.1716) -> (-6.4167, -7.8284)
  line L617 (-3.5882, -40) -> (-5.2451, -40)
  line L618 (-2.4167, -27.8284) -> (-2.4167, -26.1716)
  line L619 (-5.2451, 5) -> (-6.4167, 3.8284)
  line L620 (-6.4167, -31.1716) -> (-6.4167, -32.8284)
  line L621 (-2.4167, -2.8284) -> (-2.4167, -1.1716)
  line L622 (-5.2451, 20) -> (-6.4167, 18.8284)
  line L623 (-6.4167, 2.1716) -> (-5.2451, 1)
  line L624 (-6.4167, -1.1716) -> (-6.4167, -2.8284)
  line L625 (-6.4167, 18.8284) -> (-6.4167, 17.1716)
  line L626 (-5.2451, -29) -> (-3.5882, -29)
  line L627 (-3.5882, -49) -> (-2.4167, -47.8284)
  line L628 (-3.5882, 5) -> (-5.2451, 5)
  line L629 (-3.5882, -24) -> (-2.4167, -22.8284)
  line L630 (-6.4167, -51.1716) -> (-6.4167, -52.8284)
  line L631 (-2.4167, -6.1716) -> (-3.5882, -5)
  line L632 (-2.4167, -47.8284) -> (-2.4167, -46.1716)
  line L633 (-2.4167, -32.8284) -> (-2.4167, -31.1716)
  line L634 (-2.4167, 8.8284) -> (-3.5882, 10)
  line L635 (-6.4167, 17.1716) -> (-5.2451, 16)
  line L636 (-5.2451, -9) -> (-3.5882, -9)
  line L637 (-2.4167, -46.1716) -> (-3.5882, -45)
  line L638 (-3.5882, 16) -> (-2.4167, 17.1716)
  line L639 (-3.5882, -44) -> (-2.4167, -42.8284)
  line L640 (-5.2451, -14) -> (-3.5882, -14)
  line L641 (-3.5882, 6) -> (-2.4167, 7.1716)
  line L642 (-5.2451, -49) -> (-3.5882, -49)
  line L643 (-5.2451, -44) -> (-3.5882, -44)
  line L644 (-2.4167, -21.1716) -> (-3.5882, -20)
  line L645 (-5.2451, 1) -> (-3.5882, 1)
  line L646 (-3.5882, -4) -> (-2.4167, -2.8284)
  line L647 (-2.4167, -17.8284) -> (-2.4167, -16.1716)
  line L648 (-3.5882, -30) -> (-5.2451, -30)
  line L649 (-5.2451, -5) -> (-6.4167, -6.1716)
  line L650 (-3.5882, -19) -> (-2.4167, -17.8284)
  line L651 (-3.5882, -14) -> (-2.4167, -12.8284)
  line L652 (-6.4167, -22.8284) -> (-5.2451, -24)
  line L653 (-3.5882, -34) -> (-2.4167, -32.8284)
  line L654 (-2.4167, -31.1716) -> (-3.5882, -30)
  line L655 (-2.4167, -12.8284) -> (-2.4167, -11.1716)
  line L656 (-6.4167, -21.1716) -> (-6.4167, -22.8284)
  line L657 (-5.2451, -35) -> (-6.4167, -36.1716)
  line L658 (-5.2451, 0) -> (-6.4167, -1.1716)
  line L659 (-6.4167, -52.8284) -> (-5.2451, -54)
  line L660 (-3.5882, -10) -> (-5.2451, -10)
  line L661 (-3.5882, 1) -> (-2.4167, 2.1716)
  line L662 (-6.4167, -17.8284) -> (-5.2451, -19)
  line L663 (-6.4167, -46.1716) -> (-6.4167, -47.8284)
  line L664 (-2.4167, 17.1716) -> (-2.4167, 18.8284)
  line L665 (-5.2451, -19) -> (-3.5882, -19)
  line L666 (-5.2451, 16) -> (-3.5882, 16)
  line L667 (-5.2451, 6) -> (-3.5882, 6)
  line L668 (-5.2451, -24) -> (-3.5882, -24)
  line L669 (-5.2451, -25) -> (-6.4167, -26.1716)
  line L670 (-3.5882, -35) -> (-5.2451, -35)
  line L671 (-2.4167, 12.1716) -> (-2.4167, 13.8284)
  line L672 (-3.5882, -50) -> (-5.2451, -50)
  line L673 (-6.4167, 8.8284) -> (-6.4167, 7.1716)
  line L674 (-3.5882, 15) -> (-5.2451, 15)
  line L675 (-3.5882, -45) -> (-5.2451, -45)
  line L676 (-3.5882, 10) -> (-5.2451, 10)
  line L677 (-6.4167, -7.8284) -> (-5.2451, -9)
  line L678 (-5.2451, -50) -> (-6.4167, -51.1716)
  line L679 (-2.4167, -36.1716) -> (-3.5882, -35)
  line L680 (-6.4167, 13.8284) -> (-6.4167, 12.1716)
  line L681 (-3.5882, -9) -> (-2.4167, -7.8284)
  line L682 (-5.2451, -20) -> (-6.4167, -21.1716)
  line L683 (-5.2451, -10) -> (-6.4167, -11.1716)
  line L684 (-6.4167, -41.1716) -> (-6.4167, -42.8284)
  line L685 (-6.4167, 7.1716) -> (-5.2451, 6)
  line L686 (-5.2451, -15) -> (-6.4167, -16.1716)
  line L687 (-6.4167, -32.8284) -> (-5.2451, -34)
  line L688 (-6.4167, -42.8284) -> (-5.2451, -44)
  line L689 (-3.5882, -25) -> (-5.2451, -25)
  line L690 (-6.4167, -47.8284) -> (-5.2451, -49)
  line L691 (-2.4167, -26.1716) -> (-3.5882, -25)
  line L692 (-5.2451, -39) -> (-3.5882, -39)
  line L693 (-3.5882, 0) -> (-5.2451, 0)
  line L694 (-5.2451, 15) -> (-6.4167, 13.8284)
  line L695 (-6.4167, -37.8284) -> (-5.2451, -39)
  line L696 (-3.5882, -20) -> (-5.2451, -20)
  line L697 (-5.2451, 11) -> (-3.5882, 11)
  line L698 (-2.4167, -11.1716) -> (-3.5882, -10)
  line L699 (-6.4167, -27.8284) -> (-5.2451, -29)
  line L700 (-5.2451, 10) -> (-6.4167, 8.8284)
  line L701 (-3.5882, 11) -> (-2.4167, 12.1716)
  line L702 (-2.4167, -1.1716) -> (-3.5882, 0)
  line L703 (-3.5882, -39) -> (-2.4167, -37.8284)
  line L704 (-5.2451, -45) -> (-6.4167, -46.1716)
  line L705 (-2.4167, -22.8284) -> (-2.4167, -21.1716)
  line L706 (-6.4167, -26.1716) -> (-6.4167, -27.8284)
  line L707 (-6.4167, -16.1716) -> (-6.4167, -17.8284)
  line L708 (-3.5882, -54) -> (-2.4167, -52.8284)
  line L709 (-2.4167, -16.1716) -> (-3.5882, -15)
  line L710 (-6.4167, -11.1716) -> (-6.4167, -12.8284)
  line L711 (-5.2451, -40) -> (-6.4167, -41.1716)
  line L712 (-6.4167, -2.8284) -> (-5.2451, -4)
  line L713 (-6.4167, -12.8284) -> (-5.2451, -14)
  line L714 (-6.4167, 3.8284) -> (-6.4167, 2.1716)
  line L715 (-2.4167, -37.8284) -> (-2.4167, -36.1716)
  line L716 (-2.4167, -52.8284) -> (-2.4167, -51.1716)
  line L717 (-2.4167, -42.8284) -> (-2.4167, -41.1716)
  line L718 (-2.4167, 3.8284) -> (-3.5882, 5)
  line L719 (-3.5882, -5) -> (-5.2451, -5)
  line L720 (-2.4167, -51.1716) -> (-3.5882, -50)
  line L721 (-5.2451, -30) -> (-6.4167, -31.1716)
  line L722 (-5.2451, -4) -> (-3.5882, -4)
  line L723 (-2.4167, 7.1716) -> (-2.4167, 8.8284)
  line L724 (-5.2451, -34) -> (-3.5882, -34)
  line L725 (-3.5882, -15) -> (-5.2451, -15)
  line L726 (-2.4167, 2.1716) -> (-2.4167, 3.8284)
  line L727 (-3.5882, 20) -> (-5.2451, 20)
  line L728 (-5.2451, -54) -> (-3.5882, -54)
  line L729 (-6.4167, 12.1716) -> (-5.2451, 11)
  line L730 (-6.4167, -36.1716) -> (-6.4167, -37.8284)
  line L731 (-2.4167, -41.1716) -> (-3.5882, -40)
  line L732 (-2.4167, 13.8284) -> (-3.5882, 15)
  line L733 (-2.4167, 18.8284) -> (-3.5882, 20)
  line L734 (-2.4167, -7.8284) -> (-2.4167, -6.1716)
  line L735 (-3.5882, -29) -> (-2.4167, -27.8284)
  line L736 (-1.5, -6.1716) -> (-1.5, -7.8284)
  line L737 (1.3284, -40) -> (-0.3284, -40)
  line L738 (2.5, -27.8284) -> (2.5, -26.1716)
  line L739 (-0.3284, 5) -> (-1.5, 3.8284)
  line L740 (-1.5, -31.1716) -> (-1.5, -32.8284)
  line L741 (2.5, -2.8284) -> (2.5, -1.1716)
  line L742 (-0.3284, 20) -> (-1.5, 18.8284)
  line L743 (-1.5, 2.1716) -> (-0.3284, 1)
  line L744 (-1.5, -1.1716) -> (-1.5, -2.8284)
  line L745 (-1.5, 18.8284) -> (-1.5, 17.1716)
  line L746 (-0.3284, -29) -> (1.3284, -29)
  line L747 (1.3284, -49) -> (2.5, -47.8284)
  line L748 (1.3284, 5) -> (-0.3284, 5)
  line L749 (1.3284, -24) -> (2.5, -22.8284)
  line L750 (-1.5, -51.1716) -> (-1.5, -52.8284)
  line L751 (2.5, -6.1716) -> (1.3284, -5)
  line L752 (2.5, -47.8284) -> (2.5, -46.1716)
  line L753 (2.5, -32.8284) -> (2.5, -31.1716)
  line L754 (2.5, 8.8284) -> (1.3284, 10)
  line L755 (-1.5, 17.1716) -> (-0.3284, 16)
  line L756 (-0.3284, -9) -> (1.3284, -9)
  line L757 (2.5, -46.1716) -> (1.3284, -45)
  line L758 (1.3284, 16) -> (2.5, 17.1716)
  line L759 (1.3284, -44) -> (2.5, -42.8284)
  line L760 (-0.3284, -14) -> (1.3284, -14)
  line L761 (1.3284, 6) -> (2.5, 7.1716)
  line L762 (-0.3284, -49) -> (1.3284, -49)
  line L763 (-0.3284, -44) -> (1.3284, -44)
  line L764 (2.5, -21.1716) -> (1.3284, -20)
  line L765 (-0.3284, 1) -> (1.3284, 1)
  line L766 (1.3284, -4) -> (2.5, -2.8284)
  line L767 (2.5, -17.8284) -> (2.5, -16.1716)
  line L768 (1.3284, -30) -> (-0.3284, -30)
  line L769 (-0.3284, -5) -> (-1.5, -6.1716)
  line L770 (1.3284, -19) -> (2.5, -17.8284)
  line L771 (1.3284, -14) -> (2.5, -12.8284)
  line L772 (-1.5, -22.8284) -> (-0.3284, -24)
  line L773 (1.3284, -34) -> (2.5, -32.8284)
  line L774 (2.5, -31.1716) -> (1.3284, -30)
  line L775 (2.5, -12.8284) -> (2.5, -11.1716)
  line L776 (-1.5, -21.1716) -> (-1.5, -22.8284)
  line L777 (-0.3284, -35) -> (-1.5, -36.1716)
  line L778 (-0.3284, 0) -> (-1.5, -1.1716)
  line L779 (-1.5, -52.8284) -> (-0.3284, -54)
  line L780 (1.3284, -10) -> (-0.3284, -10)
  line L781 (1.3284, 1) -> (2.5, 2.1716)
  line L782 (-1.5, -17.8284) -> (-0.3284, -19)
  line L783 (-1.5, -46.1716) -> (-1.5, -47.8284)
  line L784 (2.5, 17.1716) -> (2.5, 18.8284)
  line L785 (-0.3284, -19) -> (1.3284, -19)
  line L786 (-0.3284, 16) -> (1.3284, 16)
  line L787 (-0.3284, 6) -> (1.3284, 6)
  line L788 (-0.3284, -24) -> (1.3284, -24)
  line L789 (-0.3284, -25) -> (-1.5, -26.1716)
  line L790 (1.3284, -35) -> (-0.3284, -35)
  line L791 (2.5, 12.1716) -> (2.5, 13.8284)
  line L792 (1.3284, -50) -> (-0.3284, -50)
  line L793 (-1.5, 8.8284) -> (-1.5, 7.1716)
  line L794 (1.3284, 15) -> (-0.3284, 15)
  line L795 (1.3284, -45) -> (-0.3284, -45)
  line L796 (1.3284, 10) -> (-0.3284, 10)
  line L797 (-1.5, -7.8284) -> (-0.3284, -9)
  line L798 (-0.3284, -50) -> (-1.5, -51.1716)
  line L799 (2.5, -36.1716) -> (1.3284, -35)
  line L800 (-1.5, 13.8284) -> (-1.5, 12.1716)
  line L801 (1.3284, -9) -> (2.5, -7.8284)
  line L802 (-0.3284, -20) -> (-1.5, -21.1716)
  line L803 (-0.3284, -10) -> (-1.5, -11.1716)
  line L804 (-1.5, -41.1716) -> (-1.5, -42.8284)
  line L805 (-1.5, 7.1716) -> (-0.3284, 6)
  line L806 (-0.3284, -15) -> (-1.5, -16.1716)
  line L807 (-1.5, -32.8284) -> (-0.3284, -34)
  line L808 (-1.5, -42.8284) -> (-0.3284, -44)
  line L809 (1.3284, -25) -> (-0.3284, -25)
  line L810 (-1.5, -47.8284) -> (-0.3284, -49)
  line L811 (2.5, -26.1716) -> (1.3284, -25)
  line L812 (-0.3284, -39) -> (1.3284, -39)
  line L813 (1.3284, 0) -> (-0.3284, 0)
  line L814 (-0.3284, 15) -> (-1.5, 13.8284)
  line L815 (-1.5, -37.8284) -> (-0.3284, -39)
  line L816 (1.3284, -20) -> (-0.3284, -20)
  line L817 (-0.3284, 11) -> (1.3284, 11)
  line L818 (2.5, -11.1716) -> (1.3284, -10)
  line L819 (-1.5, -27.8284) -> (-0.3284, -29)
  line L820 (-0.3284, 10) -> (-1.5, 8.8284)
  line L821 (1.3284, 11) -> (2.5, 12.1716)
  line L822 (2.5, -1.1716) -> (1.3284, 0)
  line L823 (1.3284, -39) -> (2.5, -37.8284)
  line L824 (-0.3284, -45) -> (-1.5, -46.1716)
  line L825 (2.5, -22.8284) -> (2.5, -21.1716)
  line L826 (-1.5, -26.1716) -> (-1.5, -27.8284)
  line L827 (-1.5, -16.1716) -> (-1.5, -17.8284)
  line L828 (1.3284, -54) -> (2.5, -52.8284)
  line L829 (2.5, -16.1716) -> (1.3284, -15)
  line L830 (-1.5, -11.1716) -> (-1.5, -12.8284)
  line L831 (-0.3284, -40) -> (-1.5, -41.1716)
  line L832 (-1.5, -2.8284) -> (-0.3284, -4)
  line L833 (-1.5, -12.8284) -> (-0.3284, -14)
  line L834 (-1.5, 3.8284) -> (-1.5, 2.1716)
  line L835 (2.5, -37.8284) -> (2.5, -36.1716)
  line L836 (2.5, -52.8284) -> (2.5, -51.1716)
  line L837 (2.5, -42.8284) -> (2.5, -41.1716)
  line L838 (2.5, 3.8284) -> (1.3284, 5)
  line L839 (1.3284, -5) -> (-0.3284, -5)
  line L840 (2.5, -51.1716) -> (1.3284, -50)
  line L841 (-0.3284, -30) -> (-1.5, -31.1716)
  line L842 (-0.3284, -4) -> (1.3284, -4)
  line L843 (2.5, 7.1716) -> (2.5, 8.8284)
  line L844 (-0.3284, -34) -> (1.3284, -34)
  line L845 (1.3284, -15) -> (-0.3284, -15)
  line L846 (2.5, 2.1716) -> (2.5, 3.8284)
  line L847 (1.3284, 20) -> (-0.3284, 20)
  line L848 (-0.3284, -54) -> (1.3284, -54)
  line L849 (-1.5, 12.1716) -> (-0.3284, 11)
  line L850 (-1.5, -36.1716) -> (-1.5, -37.8284)
  line L851 (2.5, -41.1716) -> (1.3284, -40)
  line L852 (2.5, 13.8284) -> (1.3284, 15)
  line L853 (2.5, 18.8284) -> (1.3284, 20)
  line L854 (2.5, -7.8284) -> (2.5, -6.1716)
  line L855 (1.3284, -29) -> (2.5, -27.8284)
  line L856 (3.4167, -6.1716) -> (3.4167, -7.8284)
  line L857 (6.2451, -40) -> (4.5882, -40)
  line L858 (7.4167, -27.8284) -> (7.4167, -26.1716)
  line L859 (4.5882, 5) -> (3.4167, 3.8284)
  line L860 (3.4167, -31.1716) -> (3.4167, -32.8284)
  line L861 (7.4167, -2.8284) -> (7.4167, -1.1716)
  line L862 (4.5882, 20) -> (3.4167, 18.8284)
  line L863 (3.4167, 2.1716) -> (4.5882, 1)
  line L864 (3.4167, -1.1716) -> (3.4167, -2.8284)
  line L865 (3.4167, 18.8284) -> (3.4167, 17.1716)
  line L866 (4.5882, -29) -> (6.2451, -29)
  line L867 (6.2451, -49) -> (7.4167, -47.8284)
  line L868 (6.2451, 5) -> (4.5882, 5)
  line L869 (6.2451, -24) -> (7.4167, -22.8284)
  line L870 (3.4167, -51.1716) -> (3.4167, -52.8284)
  line L871 (7.4167, -6.1716) -> (6.2451, -5)
  line L872 (7.4167, -47.8284) -> (7.4167, -46.1716)
  line L873 (7.4167, -32.8284) -> (7.4167, -31.1716)
  line L874 (7.4167, 8.8284) -> (6.2451, 10)
  line L875 (3.4167, 17.1716) -> (4.5882, 16)
  line L876 (4.5882, -9) -> (6.2451, -9)
  line L877 (7.4167, -46.1716) -> (6.2451, -45)
  line L878 (6.2451, 16) -> (7.4167, 17.1716)
  line L879 (6.2451, -44) -> (7.4167, -42.8284)
  line L880 (4.5882, -14) -> (6.2451, -14)
  line L881 (6.2451, 6) -> (7.4167, 7.1716)
  line L882 (4.5882, -49) -> (6.2451, -49)
  line L883 (4.5882, -44) -> (6.2451, -44)
  line L884 (7.4167, -21.1716) -> (6.2451, -20)
  line L885 (4.5882, 1) -> (6.2451, 1)
  line L886 (6.2451, -4) -> (7.4167, -2.8284)
  line L887 (7.4167, -17.8284) -> (7.4167, -16.1716)
  line L888 (6.2451, -30) -> (4.5882, -30)
  line L889 (4.5882, -5) -> (3.4167, -6.1716)
  line L890 (6.2451, -19) -> (7.4167, -17.8284)
  line L891 (6.2451, -14) -> (7.4167, -12.8284)
  line L892 (3.4167, -22.8284) -> (4.5882, -24)
  line L893 (6.2451, -34) -> (7.4167, -32.8284)
  line L894 (7.4167, -31.1716) -> (6.2451, -30)
  line L895 (7.4167, -12.8284) -> (7.4167, -11.1716)
  line L896 (3.4167, -21.1716) -> (3.4167, -22.8284)
  line L897 (4.5882, -35) -> (3.4167, -36.1716)
  line L898 (4.5882, 0) -> (3.4167, -1.1716)
  line L899 (3.4167, -52.8284) -> (4.5882, -54)
  line L900 (6.2451, -10) -> (4.5882, -10)
  line L901 (6.2451, 1) -> (7.4167, 2.1716)
  line L902 (3.4167, -17.8284) -> (4.5882, -19)
  line L903 (3.4167, -46.1716) -> (3.4167, -47.8284)
  line L904 (7.4167, 17.1716) -> (7.4167, 18.8284)
  line L905 (4.5882, -19) -> (6.2451, -19)
  line L906 (4.5882, 16) -> (6.2451, 16)
  line L907 (4.5882, 6) -> (6.2451, 6)
  line L908 (4.5882, -24) -> (6.2451, -24)
  line L909 (4.5882, -25) -> (3.4167, -26.1716)
  line L910 (6.2451, -35) -> (4.5882, -35)
  line L911 (7.4167, 12.1716) -> (7.4167, 13.8284)
  line L912 (6.2451, -50) -> (4.5882, -50)
  line L913 (3.4167, 8.8284) -> (3.4167, 7.1716)
  line L914 (6.2451, 15) -> (4.5882, 15)